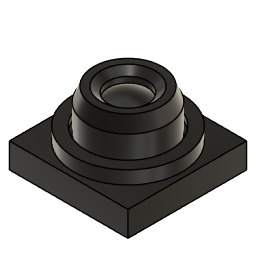
smart-sentry (Autodesk Fusion 360 archive; units mm, degrees)
design "OV3660"
Autodesk Fusion 360 part; units mm, degrees
sketch "Boceto1" plane through (0, 0, 0) normal (0, 0, 1) x (1, 0, 0)
  line L0 (-4.5, 4.5) -> (4.5, 4.5)
  line L1 (4.5, 4.5) -> (4.5, -4.5)
  line L2 (4.5, -4.5) -> (-4.5, -4.5)
  line L3 (-4.5, -4.5) -> (-4.5, 4.5)
  line L4 (-4.5, 0) -> (4.5, 0) construction
  circle A0 centre (0, 0) radius 4.1
  dimension "d1" = 9
  dimension "d3" = 8.2
  constraint horizontal L0
  constraint vertical L1
  constraint horizontal L2
  constraint vertical L3
  constraint equal L0 L1
  constraint midpoint L3 L4.start
  constraint midpoint L1 L4.end
  constraint midpoint A0.centre L4
  constraint coincident A0.centre origin
  measures "d1" distance of L0.start L0.end
  measures "d3" diameter of A0
extrude "Extruir1" add sketch "Boceto1" along normal blind 1.9 contours L0 L1 L2 L3 | A0
sketch "Boceto2" plane through (0, 0, 0) normal (0, 1, 0) x (1, 0, 0)
  line L0 (0, -5.0873) -> (0, 0)
  line L1 (-4.1, -1.9) -> (-4.1, -2.9)
  line L2 (-4.1, -2.9) -> (-3.2097, -2.9)
  line L3 (-3.2097, -2.9) -> (-3.2097, -2.4)
  line L4 (-3.2097, -2.4) -> (-3, -2.4)
  line L5 (-3, -2.4) -> (-3, -4.4695)
  line L6 (-3, -4.4695) -> (-2.5849, -5.5)
  line L7 (-2.5849, -5.5) -> (-2.0466, -5.5)
  line L8 (-4.1, -1.9) -> (0, -1.9)
  line L9 (-4.1, 0) -> (4.1, 0) construction
  line L10 (-2.0466, -5.5) -> (-1.5, -5.087)
  line L11 (-1.5, -5.087) -> (-1.5, -4.6497)
  arc A0 (-1.5, -4.6497) -> (0, -5.0873) centre (0, -2.2972) ccw
  line L12 (0, -5.0873) -> (0.6865, -5.0873) construction
  line L13 (0, -1.9) -> (0, -5.0873)
  dimension "d6" = 1.9
  dimension "d8" = 3.6
  dimension "d9" = 1
  dimension "d10" = 6
  dimension "d11" = 3
  constraint coincident L0.end origin
  constraint vertical L0
  constraint vertical L1
  constraint perpendicular L1 L2
  constraint perpendicular L2 L3
  constraint perpendicular L3 L4
  constraint perpendicular L4 L5
  constraint perpendicular L5 L7
  constraint coincident L0 L8.end
  constraint perpendicular L0 L8
  constraint coincident L1 L9.start
  constraint vertical L11
  constraint coincident L0 A0.end
  constraint tangent A0 L12
  constraint horizontal L12
  measures "d6" distance of L0.end L8
  measures "d8" distance of L7 L8
  measures "d9" distance of L1.start L1.end
revolve "Revolución1" add sketch "Boceto2" angle 360 about axis through (0, 0, 5.0873) along (0, 0, -1)

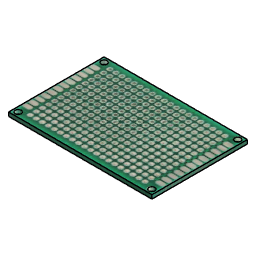
design "pcb"
Autodesk Fusion 360 part; units mm, degrees
sketch "Boceto1" plane through (0, 0, 0) normal (0, 0, 1) x (1, 0, 0)
  line L0 (-30, 20) -> (30, 20)
  line L1 (30, 20) -> (30, -20)
  line L2 (30, -20) -> (-30, -20)
  line L3 (-30, -20) -> (-30, 20)
  line L4 (-30, 0) -> (30, 0) construction
  circle A0 centre (28, -18) radius 1.27
  line L5 (0, 0) -> (0, -20) construction
  circle A1 centre (-28, -18) radius 1.27
  circle A2 centre (28, 18) radius 1.27
  circle A3 centre (-28, 18) radius 1.27
  dimension "d1" = 40
  dimension "d2" = 60
  dimension "d5" = 2.54
  dimension "d6" = 56
  dimension "d7" = 36
  constraint horizontal L0
  constraint vertical L1
  constraint horizontal L2
  constraint vertical L3
  constraint coincident L3 L4.start
  constraint coincident L1 L4.end
  constraint perpendicular L1 L4
  constraint midpoint L5.start L4
  constraint midpoint L3 L4.start
  constraint coincident L5.start origin
  constraint midpoint L2 L5.end
  constraint symmetric A0 L5 A1
  constraint symmetric L4 A0 A2
  constraint symmetric L4 A1 A3
  measures "d1" distance of L0.start L2.end
  measures "d2" distance of L0.start L0.end
  measures "d5" diameter of A0
  measures "d6" distance of A0.centre A1.centre
  measures "d7" distance of A0.centre A2.centre
extrude "Extruir1" add sketch "Boceto1" along normal blind 1.6

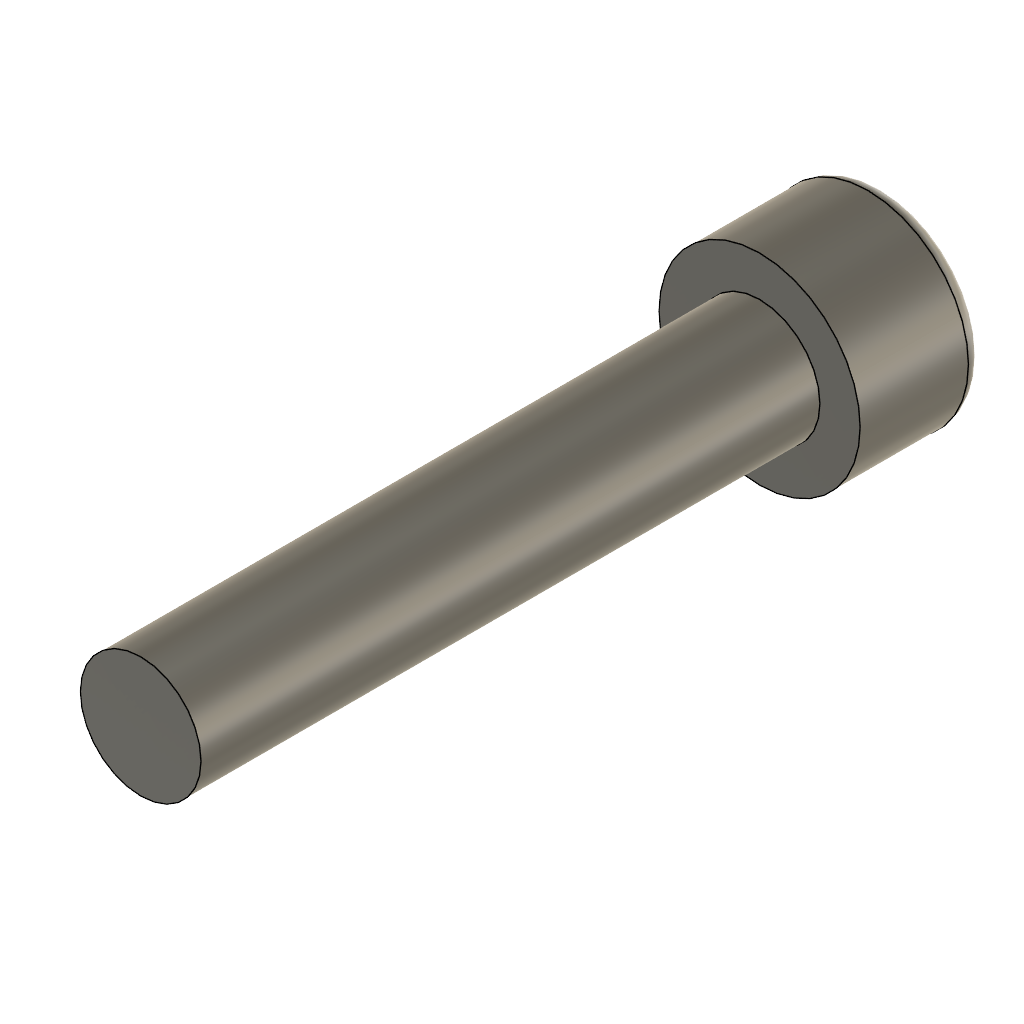
design "M8-40 allen"
Autodesk Fusion 360 part; units mm, degrees
sketch "Boceto1" plane through (0, 0, 0) normal (0, 0, 1) x (1, 0, 0)
  line L0 (0, 8) -> (-6.5, 8)
  line L1 (-6.5, 8) -> (-6.5, 0)
  line L2 (-6.5, 0) -> (-3.9, 0)
  line L3 (-3.9, 0) -> (-3.9, -40)
  line L4 (-3.9, -40) -> (0, -40)
  line L5 (0, -40) -> (0, 8)
  dimension "d1" = 7.8
  dimension "d2" = 13
  dimension "d3" = 8
  dimension "d4" = 40
  constraint horizontal L0
  constraint perpendicular L0 L1
  constraint perpendicular L1 L2
  constraint perpendicular L0 L3
  constraint perpendicular L1 L4
  constraint coincident origin L2
  constraint coincident origin L5
  constraint vertical L5
  measures "d3" distance of L0.end L1.end
  measures "d4" distance of L2.end L3.end
revolve "Revolución1" add sketch "Boceto1" angle 360 about axis through (0, -40, 0) along (0, 1, 0)
sketch "Boceto2" plane through (0, 0, 0) normal (0, 1, 0) x (1, 0, 0)
  line L0 (1.7321, 3) -> (-1.7321, 3)
  line L1 (-1.7321, 3) -> (-3.4641, 0)
  line L2 (-3.4641, 0) -> (-1.7321, -3)
  line L3 (-1.7321, -3) -> (1.7321, -3)
  line L4 (1.7321, -3) -> (3.4641, 0)
  line L5 (3.4641, 0) -> (1.7321, 3)
  dimension "d6" = 6
  constraint horizontal L0
  measures "d6" distance of L1 L4
extrude "Extruir1" cut sketch "Boceto2" along normal through all from surface at 3
fillet "Empalme1" radius 1 1 edges at (-6.0601, 8, 2.3505)

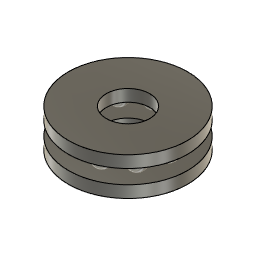
design "bearing axial"
Autodesk Fusion 360 part; units mm, degrees
sketch "Sketch1" plane through (0, 0, 0) normal (0, 1, 0) x (1, 0, 0)
  line L0 (-4, -7) -> (-11, -7)
  line L1 (-11, -7) -> (-11, -4.8)
  line L2 (-11, -4.8) -> (-4, -4.8)
  line L3 (-4, -4.8) -> (-4, -7)
  line L4 (-11, -2.2) -> (-4.1, -2.2)
  line L5 (-4.1, -2.2) -> (-4.1, 0)
  line L6 (-4.1, 0) -> (-11, 0)
  line L7 (-11, 0) -> (-11, -2.2)
  circle A0 centre (-7.5, -3.5) radius 1.6
  line L8 (0, 0) -> (0, -64)
  line L9 (-7.5, 0) -> (-7.5, -7) construction
  dimension "d13" = 3.2
  dimension "d14" = 2.2
  dimension "d15" = 22
  dimension "d16" = 8
  dimension "d17" = 8.2
  dimension "d18" = 7
  constraint horizontal L0
  constraint vertical L1
  constraint horizontal L2
  constraint vertical L3
  constraint horizontal L4
  constraint vertical L5
  constraint horizontal L6
  constraint vertical L7
  constraint equal L1 L7
  constraint coincident L8.start origin
  constraint perpendicular L6 L8
  constraint vertical L1.end L4.start
  constraint midpoint L0 L9.end
  constraint vertical L9
  constraint midpoint A0.centre L9
  constraint coincident L6 L9.start
  constraint horizontal L8.start L5.end
  measures "d13" diameter of A0
  measures "d14" distance of L0.end L1.end
  measures "d18" distance of L0 L6
revolve "Revolve2" add sketch "Sketch1" angle 360 about axis through (0, 0, 0) along (0, 0, 1) contours L0 L1 L2 L3 A0 | L2 A0 | L4 A0 | L4 L5 L6 L7 A0 makes body 1 at (-8.6438, 0.7502, 2.2) makes body 2 at (-8.6257, 0.5465, 7)
sketch "Sketch2" plane through (0, 0, 0) normal (0, 1, 0) x (1, 0, 0)
  line L0 (-7.5, 0) -> (-7.5, -7)
  arc A0 (-7.5, -1.9) -> (-7.5, -5.1) centre (-7.5, -3.5) ccw
  point P0 (-7.5, -3.5)
  point P1 (-7.5, 0)
  point P2 (-7.5, -7)
  constraint coincident P0 A0.centre
  constraint coincident P1 L0.start
  constraint coincident P2 L0.end
  constraint coincident L0 A0.end
  constraint coincident L0 A0.start
revolve "Revolve3" add sketch "Sketch2" angle 360 about axis through (-7.5, 0, 0) along (0, 0, 1) separate body makes body 3
pattern_circular "C-Pattern1" count 10 over 360 about axis through (0, 0, 0) along (0, 0, 1) of bodies 3 makes body 4 at (-7.0725, -5.606, 3.1595) makes body 5 at (-2.4267, -8.6925, 3.1595) makes body 6 at (3.1461, -8.4587, 3.1595) makes body 7 at (7.5171, -4.994, 3.1595) makes body 8 at (9.0169, 0.3782, 3.1595) makes body 9 at (7.0725, 5.606, 3.1595) makes body 10 at (2.4267, 8.6925, 3.1595) makes body 11 at (-3.1461, 8.4587, 3.1595) makes body 12 at (-7.5171, 4.994, 3.1595)

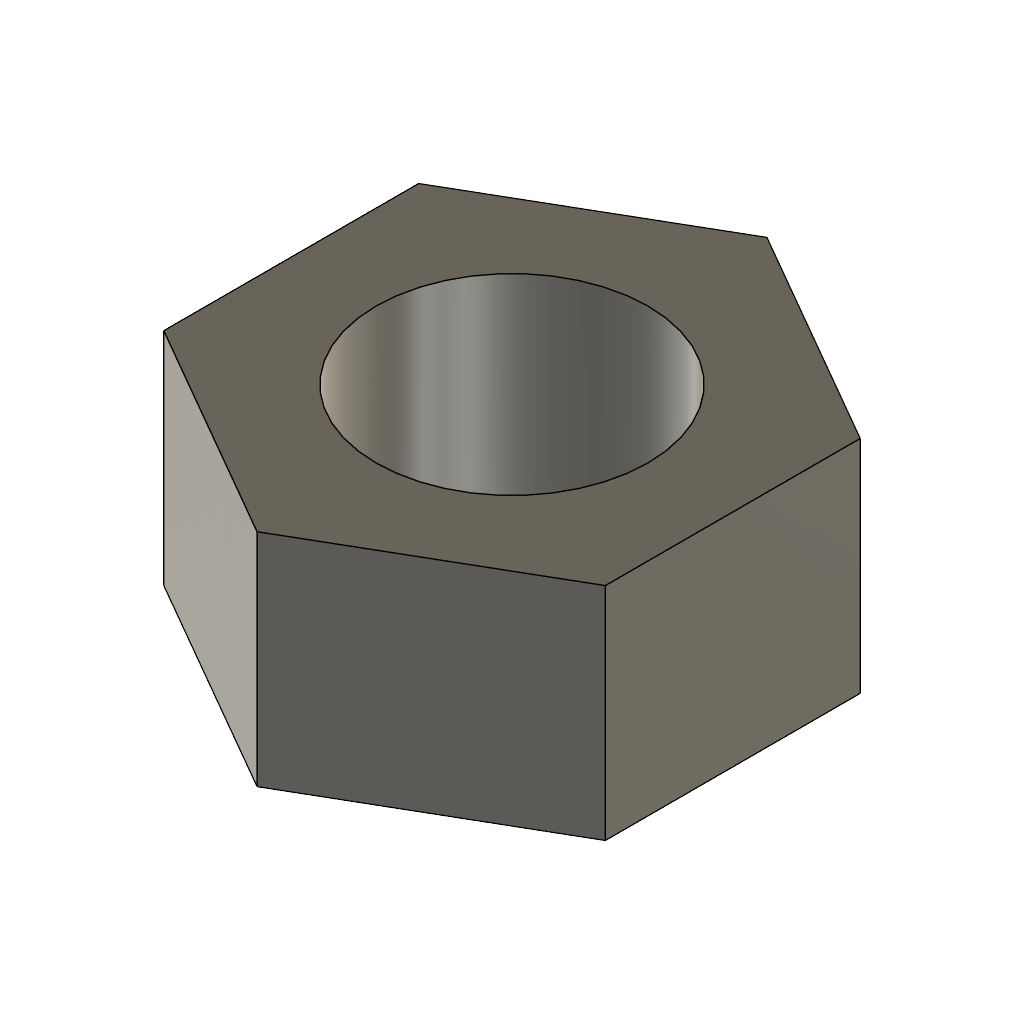
design "tuerca M8"
Autodesk Fusion 360 part; units mm, degrees
sketch "Boceto1" plane through (0, 0, 0) normal (0, 0, 1) x (1, 0, 0)
  line L0 (6.5, 3.7528) -> (0, 7.5056)
  line L1 (0, 7.5056) -> (-6.5, 3.7528)
  line L2 (-6.5, 3.7528) -> (-6.5, -3.7528)
  line L3 (-6.5, -3.7528) -> (0, -7.5056)
  line L4 (0, -7.5056) -> (6.5, -3.7528)
  line L5 (6.5, -3.7528) -> (6.5, 3.7528)
  circle A0 centre (0, 0) radius 4
  dimension "d1" = 13
  dimension "d2" = 8
  constraint coincident A0.centre origin
  constraint vertical L2
  measures "d1" distance of L2 L5
  measures "d2" diameter of A0
extrude "Extruir1" add sketch "Boceto1" along normal blind 6.5

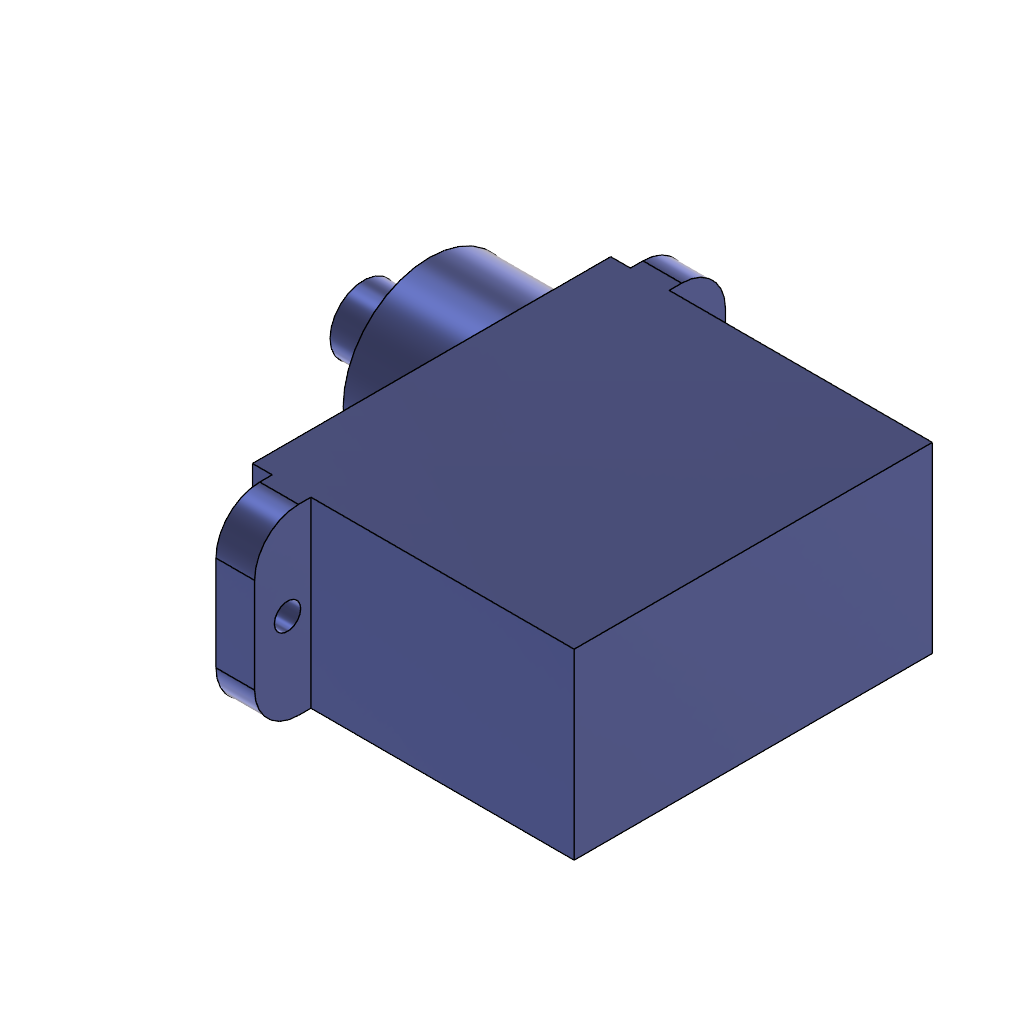
design "servo mf90"
Autodesk Fusion 360 part; units mm, degrees
sketch "Boceto1" plane through (0, 0, 0) normal (0, 0, 1) x (1, 0, 0)
  line L0 (0, 5.9) -> (28.5, 5.9)
  line L1 (28.5, 5.9) -> (28.5, -18.6)
  line L2 (28.5, -18.6) -> (6.5, -18.6)
  line L3 (6.5, -6.35) -> (28.5, -6.35) construction
  line L4 (0, 5.9) -> (0, -5.9)
  line L5 (0, -5.9) -> (6.5, -5.9)
  line L6 (6.5, -5.9) -> (6.5, -18.6)
  line L7 (6.5, -5.9) -> (6.5, 5.9)
  line L8 (0, 0) -> (-4.5, 0) construction
  line L9 (-4.5, 2.3) -> (0, 2.3)
  line L10 (0, 2.3) -> (0, -2.3)
  line L11 (0, -2.3) -> (-4.5, -2.3)
  line L12 (-4.5, -2.3) -> (-4.5, 2.3)
  line L13 (10.5, 9.75) -> (10.5, -22.45)
  line L14 (7.85, 9.75) -> (7.85, -22.45)
  line L15 (7.85, 9.75) -> (10.5, 9.75)
  line L16 (7.85, -22.45) -> (10.5, -22.45)
  point P0 (10.5, -6.35)
  dimension "d5" = 24.5
  dimension "d8" = 11.8
  dimension "d9" = 4.5
  dimension "d10" = 4.6
  dimension "d13" = 32.2
  dimension "d14" = 2.65
  dimension "d27" = 18
  dimension "d28" = 15
  dimension "d29" = 22
  constraint horizontal L0
  constraint vertical L1
  constraint horizontal L2
  constraint midpoint L1 L3.end
  constraint horizontal L3
  constraint perpendicular L0 L4
  constraint perpendicular L4 L5
  constraint vertical L6
  constraint coincident L0 L7.end
  constraint perpendicular L0 L7
  constraint midpoint L4 L8.start
  constraint perpendicular L4 L8
  constraint horizontal L9
  constraint vertical L10
  constraint horizontal L11
  constraint vertical L12
  constraint midpoint L8.end L12
  constraint coincident L4 L10.end
  constraint coincident L8.start origin
  constraint coincident L3.start L6
  constraint perpendicular L2 L13
  constraint midpoint L13 P0
  constraint coincident L3 P0
  constraint perpendicular L13 L15
  constraint perpendicular L13 L16
  measures "d5" distance of L0 L2
  measures "d8" distance of L0.start L4.end
  measures "d9" distance of L10.end L11.end
  measures "d10" distance of L9.start L11.end
  measures "d13" distance of L13.start L13.end
  measures "d27" distance of L1 L13
  measures "d28" distance of L12 L13
  measures "d29" distance of L1 L6
extrude "Extruir1" add sketch "Boceto1" along normal mid plane 12.5 contours L0 L2 L6 L7 L14 | L0 L13 L14 L15 | L0 L2 L13 L14 | L0 L1 L2 L13 | L2 L13 L14 L16
sketch "Boceto2" plane through (0, 0, 0) normal (1, 0, 0) x (0, 1, 0)
  circle A0 centre (0, 0) radius 5.9
  circle A1 centre (0, 0) radius 2.3
  point P0 (-5.9, 0)
  point P1 (-2.3, 0)
  point P2 (-5.9, 0)
  constraint coincident A0.centre A1.centre
  constraint concentric A0 A1
  constraint coincident A0 P2
  constraint coincident A1 P1
extrude "Extruir2" add sketch "Boceto2" along normal up to surface (6.5 mm away) contours A0 | A1
extrude "Extruir3" add sketch "Boceto2" against normal up to surface (4.5 mm away) contours A1
sketch "Boceto3" plane through (0, 0, 0) normal (1, 0, 0) x (0, 1, 0)
  line L0 (-20.2, 0) -> (7.5, 0) construction
  circle A0 centre (-20.2, 0) radius 0.9
  circle A1 centre (7.5, 0) radius 0.9
  point P0 (-6.35, 0)
  dimension "d21" = 27.7
  dimension "d22" = 1.8
  constraint horizontal L0
  constraint coincident origin L0
  constraint midpoint L0 P0
  constraint coincident L0.start A0.centre
  constraint coincident L0.end A1.centre
  constraint equal A0 A1
  measures "d21" distance of L0.start L0.end
  measures "d22" diameter of A0
extrude "Extruir4" cut sketch "Boceto3" along normal through all
fillet "Empalme1" radius 3 4 edges at (9.175, -22.45, -6.25) (9.175, -22.45, 6.25) (9.175, 9.75, -6.25) (9.175, 9.75, 6.25)
equation "L = 23 mm"
equation "An = 12.5 mm"
equation "Al = 21.8 mm"
equation "d15 = An"
equation "d21 = screw_dist"
equation "screw_dist = 27.7 mm"

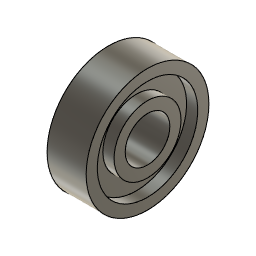
design "bearing 22-8-7"
Autodesk Fusion 360 part; units mm, degrees
sketch "Sketch1" plane through (0, 0, 0) normal (0, 1, 0) x (1, 0, 0)
  line L0 (-5, 0) -> (5, 0)
  line L1 (0, 8.5) -> (0, 0)
  line L2 (-3.5, 4) -> (-3.5, 6)
  line L3 (-3.5, 6) -> (-1.5, 6)
  line L4 (-1.5, 6) -> (-1.5, 9)
  line L5 (-1.5, 9) -> (-3.5, 9)
  line L6 (-3.5, 9) -> (-3.5, 11)
  line L7 (3.5, 9) -> (3.5, 11)
  line L8 (1.5, 9) -> (3.5, 9)
  line L9 (1.5, 6) -> (1.5, 9)
  line L10 (3.5, 6) -> (1.5, 6)
  line L11 (3.5, 4) -> (3.5, 6)
  line L12 (-3.5, 11) -> (3.5, 11)
  line L13 (3.5, 4) -> (-3.5, 4)
  dimension "d44" = 2
  dimension "d45" = 7
  dimension "d46" = 22
  dimension "d47" = 8
  constraint horizontal L0
  constraint coincident L1.end origin
  constraint perpendicular L0 L1
  constraint coincident L0 L1.end
  constraint perpendicular L1 L3
  constraint perpendicular L1 L5
  constraint symmetric L1 L6.end L7.end
  constraint symmetric L1 L2.start L11.start
  constraint symmetric L1 L2.end L10.start
  constraint symmetric L1 L3.end L9.start
  constraint symmetric L1 L4.end L8.start
  constraint symmetric L1 L5.end L7.start
  constraint perpendicular L2 L13
  constraint vertical L2.end L5.end
  constraint equal L2 L6
  constraint equal L2 L3
  constraint vertical L4
  measures "d44" distance of L6.end L5.end
  measures "d45" distance of L6.end L7.end
revolve "Revolve1" add sketch "Sketch1" angle 360 about axis through (-5, 0, 0) along (1, 0, 0)

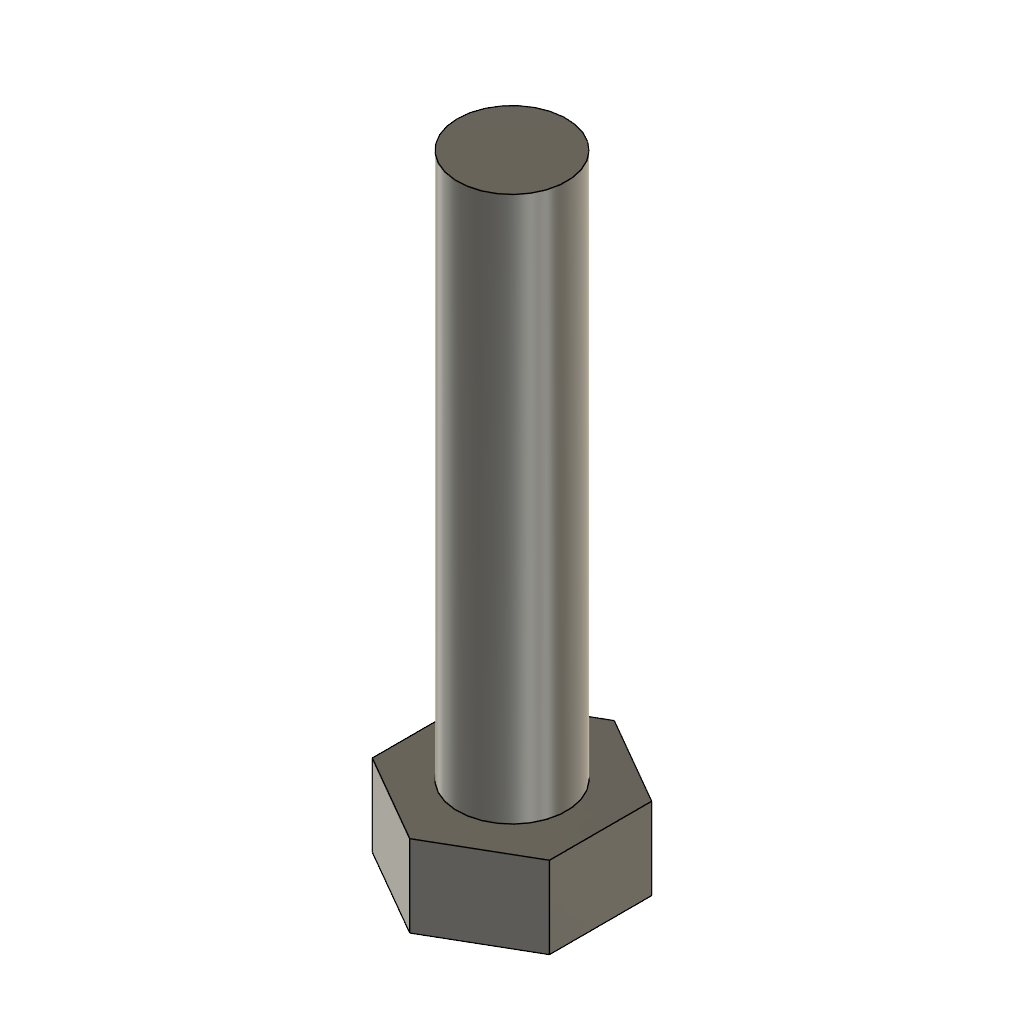
design "M8-40 hex"
Autodesk Fusion 360 part; units mm, degrees
sketch "Boceto1" plane through (0, 0, 0) normal (0, 0, 1) x (1, 0, 0)
  circle A0 centre (0, 0) radius 4
  line L0 (6.5, 3.7528) -> (0, 7.5056)
  line L1 (0, 7.5056) -> (-6.5, 3.7528)
  line L2 (-6.5, 3.7528) -> (-6.5, -3.7528)
  line L3 (-6.5, -3.7528) -> (0, -7.5056)
  line L4 (0, -7.5056) -> (6.5, -3.7528)
  line L5 (6.5, -3.7528) -> (6.5, 3.7528)
  dimension "d1" = 8
  dimension "d2" = 13
  constraint coincident A0.centre origin
  constraint vertical L2
  measures "d1" diameter of A0
  measures "d2" distance of L2 L5
extrude "Extruir1" add sketch "Boceto1" along normal blind 6 contours A0 | L0 L1 L2 L3 L4 L5
extrude "Extruir2" add sketch "Boceto1" along normal blind 40 from surface at 6 contours A0

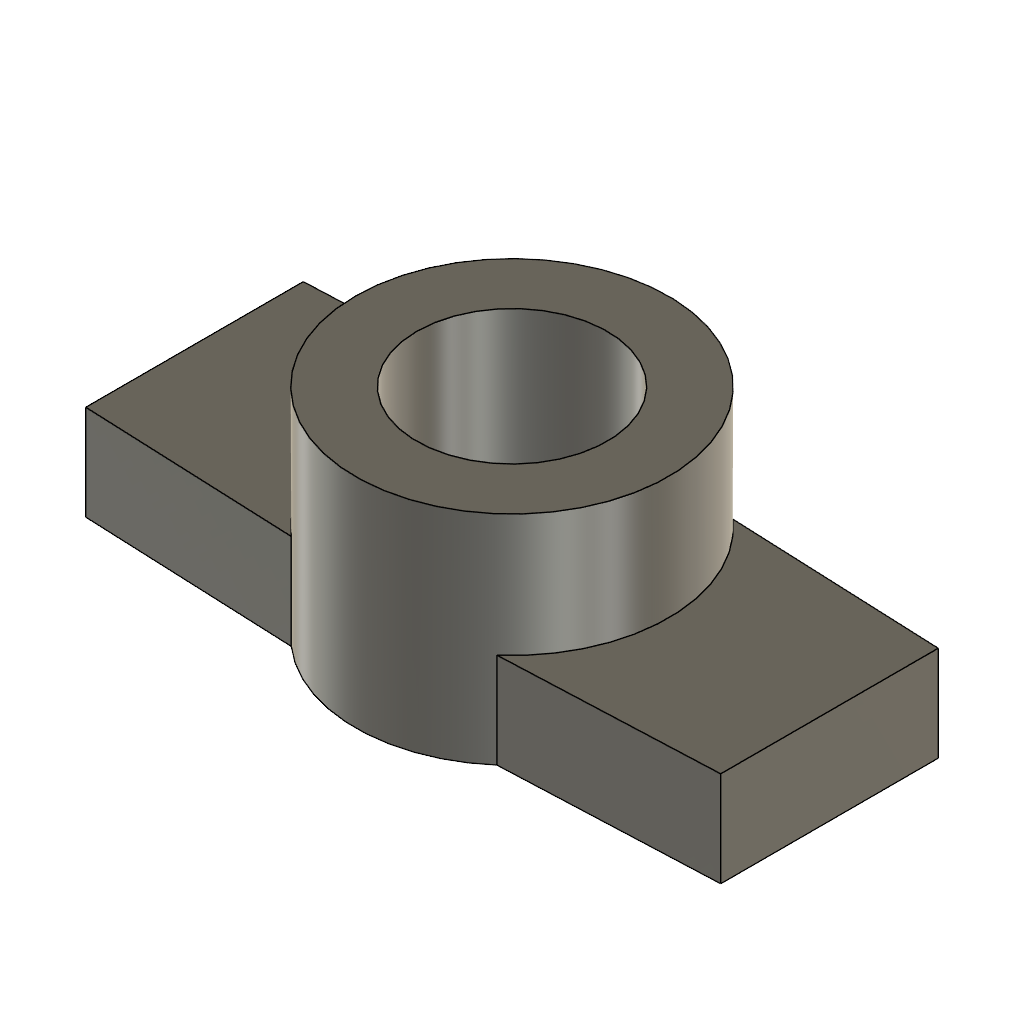
design "horn"
Autodesk Fusion 360 part; units mm, degrees
sketch "Boceto1" plane through (0, 0, 0) normal (0, 0, 1) x (1, 0, 0)
  circle A0 centre (0, 0) radius 3.45
  line L0 (7, 2.3987) -> (7, -2.3987)
  line L1 (-7, -2.3987) -> (-7, 2.3987)
  line L2 (-7, 0) -> (7, 0) construction
  line L3 (0, 1.65) -> (0, 0) construction
  circle A1 centre (0, 0) radius 1.25
  circle A2 centre (0, 0) radius 2.1
  line L4 (0, 2.6964) -> (0, -2.6964) construction
  line L5 (-7, 2.3987) -> (0, 2.6964)
  line L6 (0, 2.6964) -> (7, 2.3987)
  line L7 (7, -2.3987) -> (0, -2.6964)
  line L8 (-7, -2.3987) -> (0, -2.6964)
  line L9 (7, -2.3987) -> (15.2, -2.05) construction
  line L10 (15.2, -2.05) -> (15.2, 2.05) construction
  line L11 (15.2, 2.05) -> (7, 2.3987) construction
  line L12 (15.2, 0) -> (7, 0) construction
  line L13 (-15.2, 2.05) -> (-7, 2.3987) construction
  line L14 (-15.2, -2.05) -> (-15.2, 2.05) construction
  line L15 (-7, -2.3987) -> (-15.2, -2.05) construction
  point P0 (2.2677, 2.6)
  point P1 (2.2677, -2.6)
  dimension "d1" = 6.9
  dimension "d8" = 2.5
  dimension "d9" = 4.2
  dimension "d14" = 14
  dimension "d15" = 4.1
  dimension "d16" = 30.4
  dimension "d17" = 5.2
  constraint coincident A0.centre L3.end
  constraint vertical L0
  constraint vertical L1
  constraint midpoint L1 L2.start
  constraint midpoint L0 L2.end
  constraint midpoint L2 A0.centre
  constraint vertical L4
  constraint midpoint A0.centre L4
  constraint parallel L0 L10
  constraint collinear L7 L9
  constraint collinear L6 L11
  constraint horizontal L2
  constraint midpoint L10 L12.start
  constraint symmetric L0.start L4 L1.end
  constraint symmetric L0.end L4 L1.start
  constraint symmetric L4 L9.end L14.start
  constraint symmetric L4 L10.end L13.start
  constraint coincident L1.end L5.start
  constraint coincident A0 P0
  constraint coincident L6 P0
  constraint coincident L7 P1
  constraint coincident A0 P1
  measures "d1" diameter of A0
  measures "d8" diameter of A1
  measures "d9" diameter of A2
  measures "d14" distance of L0 L1
  measures "d15" distance of L9.end L10.end
  measures "d16" distance of L10 L14
  measures "d17" distance of P0 P1
extrude "Extruir1" add sketch "Boceto1" along normal blind 2.1 contours A0 L5 L6 L7 L8 | A0 L0 L6 L7 | A0 L5 L6 | A0 L7 L8 | A0 L1 L5 L8 | A2
extrude "Extruir2" add sketch "Boceto1" along normal blind 4.8 contours A0 L5 L6 L7 L8 | A0 L5 L6 | A0 L7 L8 | A2
extrude "Extruir3" cut sketch "Boceto1" along normal through all from surface at 1 contours A2
equation "d1 = 6.8 mm + gap * 2"
equation "d15 = 4 mm + gap * 2"
equation "d16 = 30.3 mm + gap * 2"
equation "d17 = 5.1 mm + gap * 2"
equation "gap = 0.05 mm"

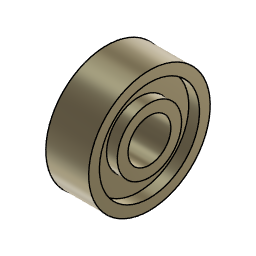
design "bearing 17-6-6"
Autodesk Fusion 360 part; units mm, degrees
sketch "Sketch1" plane through (0, 0, 0) normal (0, 1, 0) x (1, 0, 0)
  line L0 (-3, 0) -> (3, 0)
  line L1 (0, 0) -> (0, 8.5)
  line L2 (-3, 8.5) -> (3, 8.5)
  line L3 (3, 8.5) -> (3, 7)
  line L4 (3, 7) -> (1.5, 7)
  line L5 (1.5, 7) -> (1.5, 4.5)
  line L6 (1.5, 4.5) -> (3, 4.5)
  line L7 (3, 4.5) -> (3, 3)
  line L8 (3, 3) -> (-3, 3)
  line L9 (-3, 3) -> (-3, 4.5)
  line L10 (-3, 4.5) -> (-1.5, 4.5)
  line L11 (-1.5, 4.5) -> (-1.5, 7)
  line L12 (-1.5, 7) -> (-3, 7)
  line L13 (-3, 7) -> (-3, 8.5)
  dimension "d8" = 6
  dimension "d9" = 17
  dimension "d10" = 1.5
  dimension "d11" = 6
  constraint horizontal L0
  constraint perpendicular L0 L1
  constraint coincident L1.start origin
  constraint coincident L0 L1.start
  constraint horizontal L2
  constraint perpendicular L2 L3
  constraint perpendicular L3 L4
  constraint perpendicular L4 L5
  constraint perpendicular L5 L6
  constraint perpendicular L6 L7
  constraint perpendicular L1 L8
  constraint perpendicular L8 L9
  constraint perpendicular L9 L10
  constraint perpendicular L8 L11
  constraint perpendicular L11 L12
  constraint perpendicular L2 L13
  constraint symmetric L1 L7 L9
  constraint equal L9 L13
  constraint equal L7 L9
  constraint equal L3 L13
  constraint vertical L0.start L8.end
  constraint vertical L0.end L7.end
  constraint vertical L3.end L6.end
  constraint vertical L9.end L12.end
  constraint midpoint L1.end L2
  constraint equal L9 L10
  constraint equal L6 L7
  measures "d10" distance of L8.end L9.end
  measures "d11" distance of L2.start L2.end
revolve "Revolve1" add sketch "Sketch1" angle 360 about axis through (-3, 0, 0) along (1, 0, 0)
